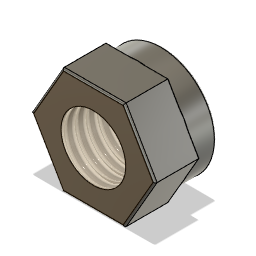
7.167.4602 - Ecrou HFR M12 (Autodesk Fusion 360 design; units mm, degrees)
Autodesk Fusion 360 part; units mm, degrees
sketch "Sketch1" plane through (0, 0, 0) normal (0, 0, 1) x (1, 0, 0)
  circle A0 centre (0, 0) radius 6
  circle A1 centre (0, 0) radius 8.5
  dimension "d1" = 12
  dimension "d2" = 2.5
  constraint coincident A0.centre A1.centre
  measures "d1" diameter of A0
extrude "Extrude1" add sketch "Sketch1" along normal blind 4
sketch "Sketch2" plane through (0, 0, 4) normal (0, 0, 1) x (1, 0, 0)
  circle A0 centre (0, 0) radius 6
  circle A1 centre (0, 0) radius 8.5
  line L0 (-4.9075, 8.5) -> (-9.815, 0)
  line L1 (-9.815, 0) -> (-4.9075, -8.5)
  line L2 (-4.9075, -8.5) -> (4.9075, -8.5)
  line L3 (4.9075, -8.5) -> (9.815, 0)
  line L4 (9.815, 0) -> (4.9075, 8.5)
  line L5 (4.9075, 8.5) -> (-4.9075, 8.5)
  circle A2 centre (0, 0) radius 6
  constraint coincident A0.centre A1.centre
  constraint tangent A1 L5
extrude "Extrude2" add sketch "Sketch2" along normal blind 7
fillet "Fillet1" radius 0.3 6 edges at (0, -8.5, 11) (-7.3612, -4.25, 11) (-7.3612, 4.25, 11) (0, 8.5, 11) (7.3612, 4.25, 11) (7.3612, -4.25, 11)
fillet "Fillet2" radius 0.1 12 edges at (-2.4537, -8.5, 4) (-6.1343, -6.375, 4) (-8.5881, -2.125, 4) (-8.5881, 2.125, 4) (-6.1343, 6.375, 4) (-2.4537, 8.5, 4) (2.4537, 8.5, 4) (6.1343, 6.375, 4) (8.5881, 2.125, 4) (8.5881, -2.125, 4) (6.1343, -6.375, 4) (2.4537, -8.5, 4)
fillet "Fillet3" radius 0.3 1 edges at (-7.9248, -3.0737, 0)
thread "Thread2" "ISO Metric profile 12.0 M12x1.75 6H" major diameter 12.2265 minor diameter 10.2735 pitch 1.75 angle 60 resizes the face on face at (5.9702, -0.5974, 3.6667)
sketch "Sketch3" plane through (0, 0, 11) normal (0, 0, 1) x (1, 0, 0)
  circle A0 centre (0, 0) radius 5.1368
  line L0 (4.7343, 8.2) -> (-4.7343, 8.2)
  line L1 (-4.7343, 8.2) -> (-9.4685, 0)
  line L2 (-9.4685, 0) -> (-4.7343, -8.2)
  line L3 (-4.7343, -8.2) -> (4.7343, -8.2)
  line L4 (4.7343, -8.2) -> (9.4685, 0)
  line L5 (9.4685, 0) -> (4.7343, 8.2)
